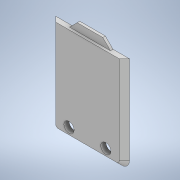
# Autodesk Inventor part: OBS-MainCase-A-004_GPS-Cover_v0.1.1
Saved by Autodesk Inventor 2021.1 (Build 251245010, 245A)
## iProperties
Created: 2021-04-10
Part Number: OBS-MainCase-A-004_GPS-Cover_v0.1.1
Material: Generisch
Document SubType Name: Modeling
Designer: hpcthobs
Density: 1 g/cm^3
Appearance: Vorgabe
Author: hpcthobs
Autodesk Inventor part; units mm, degrees
ref_plane "YZ Plane" through (0, 0, 0) normal (1, 0, 0) x (0, 1, 0)
ref_plane "XZ Plane" through (0, 0, 0) normal (0, 1, 0) x (-1, 0, 0)
ref_plane "XY Plane" through (0, 0, 0) normal (0, 0, 1) x (1, 0, 0)
sketch "Skizze1" plane through (0, 0, 0) normal (0, 0, 1) x (1, 0, 0)
  line L0 (3.4, 37.6) -> (-3, 37.6)
  line L1 (-3, 37.6) -> (-3, 3)
  arc A0 (-3, 3) -> (0, 0) centre (0, 3) ccw
  line L2 (0, 0) -> (22.8, 0)
  arc A1 (22.8, 0) -> (25.8, 3) centre (22.8, 3) ccw
  line L3 (25.8, 3) -> (25.8, 37.6)
  line L4 (25.8, 37.6) -> (19.4, 37.6)
  line L5 (19.4, 37.6) -> (16.4, 40.6)
  line L6 (16.4, 40.6) -> (6.4, 40.6)
  line L7 (6.4, 40.6) -> (3.4, 37.6)
  line L8 (-1.8, 35.6) -> (24.6, 35.6)
  line L9 (24.6, 35.6) -> (24.6, 9.2)
  line L10 (24.6, 9.2) -> (-1.8, 9.2)
  line L11 (-1.8, 9.2) -> (-1.8, 35.6)
  line L12 (24.6, 35.6) -> (-1.8, 35.6)
  line L13 (-1.8, 35.6) -> (-1.8, 9.2)
  line L14 (-1.8, 9.2) -> (24.6, 9.2)
  line L15 (24.6, 9.2) -> (24.6, 35.6)
  line L16 (24.6, 35.6) -> (-1.8, 35.6)
  line L17 (-3, 37.6) -> (3.4, 37.6)
  line L18 (-3, 3) -> (-3, 37.6)
  arc A2 (-3, 3) -> (0, 0) centre (0, 3) ccw
  line L19 (22.8, 0) -> (0, 0)
  arc A3 (22.8, 0) -> (25.8, 3) centre (22.8, 3) ccw
  line L20 (25.8, 37.6) -> (25.8, 3)
  line L21 (19.4, 37.6) -> (25.8, 37.6)
  line L22 (19.4, 37.6) -> (16.4, 40.6)
  line L23 (16.4, 40.6) -> (6.4, 40.6)
  line L24 (6.4, 40.6) -> (3.4, 37.6)
  circle A4 centre (4.1926, 4.6) radius 2
  line L25 (11.4, 35.6) -> (11.4, 0)
  circle A5 centre (18.6074, 4.6) radius 2
  point P0 (-3, 37.6)
  point P1 (-3, 3)
  point P2 (0, 0)
  constraints: 52 end point, 8 point on circle, 6 centre point
extrude "Extrusion1" add sketch "Skizze1" along normal blind 2 contours L7 L6 L5 L4 L3 A1 L2 A0 L1 L0 | L8 L25 L10 L11 | L8 L9 L10 L25
chamfer "Fase1" distance 2 angle 45 5 edges at (25.8, 20.3, 2) (24.9213, 0.8787, 2) (11.4, 0, 2) (-2.1213, 0.8787, 2) (-3, 20.3, 2)
sketch "Skizze2" plane through (0, 0, 2) normal (0, 0, 1) x (1, 0, 0)
  line L0 (-1, 3) -> (-1, 37.6) projected
  arc A0 (-1, 3) -> (0, 2) centre (0, 3) ccw projected
  line L1 (22.8, 2) -> (0, 2) projected
  arc A1 (22.8, 2) -> (23.8, 3) centre (22.8, 3) ccw projected
  line L2 (23.8, 37.6) -> (23.8, 3) projected
  line L3 (23.8, 37.6) -> (19.4, 37.6) projected
  line L4 (19.4, 37.6) -> (16.4, 40.6) projected
  line L5 (16.4, 40.6) -> (6.4, 40.6) projected
  line L6 (6.4, 40.6) -> (3.4, 37.6) projected
  line L7 (3.4, 37.6) -> (-1, 37.6) projected
  line L8 (6.4, 40.6) -> (3.4, 37.6) projected
  line L9 (3.4, 37.6) -> (19.4, 37.6)
  point P0 (0, 0)
  constraints: 2 end point, 1 horizontal
extrude "Extrusion2" cut sketch "Skizze2" against normal blind 1 contours L6 L5 L4 L9
